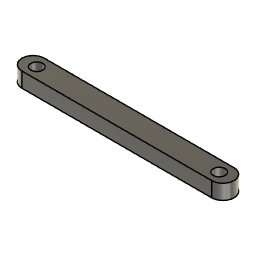
fixer_1 (Autodesk Fusion 360 design; units mm, degrees)
Autodesk Fusion 360 part; units mm, degrees
sketch "Esboço1" plane through (0, 0, 0) normal (0, 0, 1) x (1, 0, 0)
  line L0 (18.163, 18) -> (75.223, 18)
  line L1 (75.223, 18) -> (75.223, 12)
  line L2 (75.223, 12) -> (18.163, 12)
  line L3 (18.163, 12) -> (18.163, 18)
  circle A0 centre (22.163, 15) radius 1.6
  circle A1 centre (71.223, 15) radius 1.6
  dimension "d2" = 3.2
  dimension "d3" = 3.2
  dimension "d4" = 49.06
  dimension "d5" = 4
  dimension "d6" = 4
  dimension "d13" = 6
  dimension "d14" = 3
  constraint horizontal L0
  constraint vertical L1
  constraint horizontal L2
  constraint vertical L3
  measures "d2" diameter of A0
  measures "d3" diameter of A1
  measures "d4" distance of A0.centre A1.centre
  measures "d5" distance of L3 A0.centre
  measures "d6" distance of L1 A1.centre
  measures "d13" distance of L0.start L2.end
  measures "d14" distance of L0 A0.centre
extrude "Extrusão1" add sketch "Esboço1" along normal blind 4
fillet "Arredondamento3" radius 3 2 edges at (18.163, 18, 2) (18.163, 12, 2)
fillet "Arredondamento4" radius 3 2 edges at (75.223, 18, 2) (75.223, 12, 2)
scale "Escala1" factor 0.7 about (20.563, 15, 0) bodies 1
scale "Escala2" factor 1.14 about (20.983, 17.1, 2.8) bodies 1
